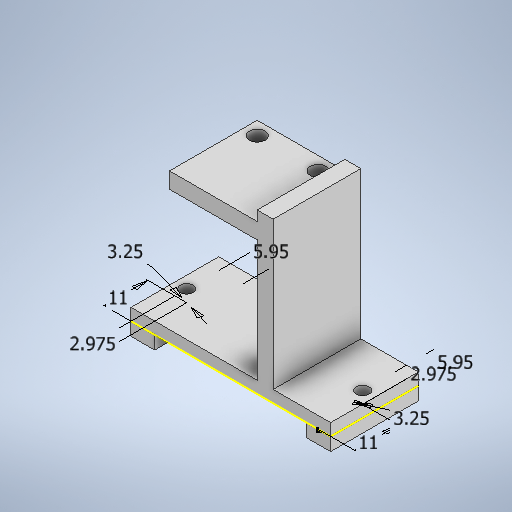
# Autodesk Inventor part: IMU_shin_mount
Saved by Autodesk Inventor 2025.2 (Build 292293000, 293)
## iProperties
Created: 2025-01-16
Part Number: IMU_shin_mount
Material: Generic
Document SubType Name: Modeling
Designer: email
Density: 1 g/cm^3
Appearance: Default
Author: email
Autodesk Inventor part; units mm, degrees
ref_plane "YZ Plane" through (0, 0, 0) normal (1, 0, 0) x (0, 1, 0)
ref_plane "XZ Plane" through (0, 0, 0) normal (0, 1, 0) x (-1, 0, 0)
ref_plane "XY Plane" through (0, 0, 0) normal (0, 0, 1) x (1, 0, 0)
sketch "Sketch1" plane through (0, 0, 0) normal (0, 0, 1) x (1, 0, 0)
  line L0 (0, 0) -> (50.1, 0)
  line L1 (50.1, 0) -> (50.1, 3)
  line L2 (50.1, 3) -> (0, 3)
  line L3 (0, 3) -> (0, 0)
  line L4 (35.6718, 0) -> (31.6718, 0)
  line L5 (31.6718, 0) -> (31.6718, 40)
  line L6 (31.6718, 40) -> (35.6718, 40)
  line L7 (35.6718, 40) -> (35.6718, 0)
  line L8 (31.6718, 37.5) -> (9.6718, 37.5)
  line L9 (9.6718, 37.5) -> (9.6718, 33.5)
  line L10 (9.6718, 33.5) -> (31.6718, 33.5)
  line L11 (31.6718, 33.5) -> (31.6718, 37.5)
  line L12 (5.95, 0) -> (44.15, 0)
  line L13 (44.15, 0) -> (44.15, 3)
  line L14 (44.15, 3) -> (5.95, 3)
  line L15 (5.95, 3) -> (5.95, 0)
  point P0 (35.6718, 3)
  point P1 (31.6718, 3)
  dimension "d0" = 50.1
  dimension "d1" = 3
  dimension "d2" = 40
  dimension "d3" = 22
  dimension "d4" = 4
  dimension "d5" = 2.5
  dimension "d6" = 38.2
  dimension "d7" = 5.95
  dimension "d30" = 4
  constraints: 32 end point, 8 parallel, 4 horizontal, 4 perpendicular, 4 point on line
  measures "d0" distance of L1.end L2.end
  measures "d1" distance of L2.end L0.start
  measures "d2" distance of L6.end L4.start
  measures "d3" distance of L9.end L10.end
  measures "d4" distance of L8.end L9.end
  measures "d5" distance between parallel lines of L6 L8
  measures "d6" distance between parallel lines of L15 L13
  measures "d7" distance between parallel lines of L3 L15
  measures "d30" distance of L5.end L6.end
extrude "Extrusion1" add sketch "Sketch1" along normal blind 22
sketch "Sketch2" plane through (0, 0, 0) normal (0, -1, 0) x (1, 0, 0)
  line L0 (50.1, 0) -> (50.1, 22) projected
  line L1 (0, 22) -> (50.1, 22) projected
  line L2 (50.1, 0) -> (44.15, 0)
  line L3 (44.15, 0) -> (44.15, 22)
  line L4 (44.15, 22) -> (50.1, 22)
  line L5 (50.1, 22) -> (50.1, 0)
  line L6 (0, 0) -> (5.95, 0)
  line L7 (5.95, 0) -> (5.95, 22)
  line L8 (5.95, 22) -> (0, 22)
  line L9 (0, 22) -> (0, 0)
  circle A0 centre (47.125, 11) radius 1.625
  circle A1 centre (2.975, 11) radius 1.625
  point P0 (47.125, 22)
  point P1 (0, 11)
  dimension "d10" = 5.95
  dimension "d11" = 5.95
  dimension "d14" = 3.25
  dimension "d15" = 3.25
  dimension "d16" = 2.975
  dimension "d17" = 11
  dimension "d18" = 2.975
  dimension "d19" = 11
  constraints: 16 end point, 4 parallel, 2 centre point, 2 horizontal, 2 midpoint, 2 perpendicular, 2 point on line
  measures "d10" distance between parallel lines of L0 L3
  measures "d11" distance between parallel lines of L9 L7
  measures "d14" diameter of A0
  measures "d15" diameter of A1
  measures "d16" distance from line of L0 A0.centre
  measures "d17" distance of point (47.125, 22) A0.centre
  measures "d18" distance of point (0, 11) A1.centre
  measures "d19" distance from line of L1 A1.centre
extrude "Extrusion2" add sketch "Sketch2" along normal blind 3.3 contours L2 L3 L1 L0 | L7 L6 L9 L1 | A0 | A1
extrude "Extrusion3" cut sketch "Sketch2" along normal through all both and the other way through all contours A0 | A1
sketch "Sketch3" plane through (9.6718, 37.5, 0) normal (0, 1, 0) x (1, 0, 0)
  circle A0 centre (18.65, -18.65) radius 2
  circle A1 centre (18.65, -3.35) radius 2
  line L0 (22, 0) -> (22, -22) projected
  line L1 (22, -22) -> (-9.6718, -22) projected
  line L2 (22, 0) -> (0, 0) projected
  circle A2 centre (3.35, -3.35) radius 2
  line L3 (0, 0) -> (0, -22) projected
  point P0 (-9.6718, 0)
  point P1 (11, 0)
  dimension "d22" = 3.35
  dimension "d23" = 4
  dimension "d24" = 4
  dimension "d25" = 15.3
  dimension "d26" = 3.35
  dimension "d31" = 15.3
  dimension "d32" = 4
  dimension "d33" = 3.35
  dimension "d34" = 3.35
  constraints: 3 centre point, 1 midpoint, 1 vertical alignment
  measures "d22" distance from line of L0 A0.centre
  measures "d23" diameter of A0
  measures "d24" diameter of A1
  measures "d25" distance of A1.centre A0.centre
  measures "d26" distance from line of L1 A0.centre
  measures "d31" distance of A1.centre A2.centre
  measures "d32" diameter of A2
  measures "d33" distance from line of L0 A1.centre
  measures "d34" distance from line of L3 A2.centre
extrude "Extrusion4" cut sketch "Sketch3" against normal blind 10 contours A1 | A2
equation "\"d7\" = -0.5 * d6 + 0.5 * d0"
body "Solid1"
